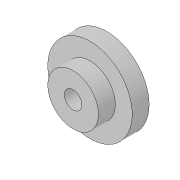
# Autodesk Inventor part: T-Spacer 3 of 32 inch
Saved by Autodesk Inventor 2018.3 (Build 223284000, 284)
## iProperties
Created: 2019-03-14
Part Number: T-Spacer 3 of 32 inch
Material: Generic
Document SubType Name: Modeling
Designer: aye06091
Mass: 0.797081 g
Surface Area: 6.96192 cm^2
Volume: 0.797081 cm^3
Density: 1 g/cm^3
Appearance: Default
Author: aye06091
Autodesk Inventor part; units mm, degrees
ref_plane "YZ Plane" through (0, 0, 0) normal (1, 0, 0) x (0, 1, 0)
ref_plane "XZ Plane" through (0, 0, 0) normal (0, 1, 0) x (-1, 0, 0)
ref_plane "XY Plane" through (0, 0, 0) normal (0, 0, 1) x (1, 0, 0)
sketch "Sketch4" plane through (0, 0, 0) normal (0, 0, 1) x (1, 0, 0)
  circle A0 centre (0, 0) radius 1.651
  circle A1 centre (0, 0) radius 4.7498
  dimension "d9" = 3.302
  dimension "d16" = 9.4996
  constraints: 2 centre point, 2 coincident
  measures "d9" diameter of A0
  measures "d16" diameter of A1
extrude "Extrusion4" add sketch "Sketch4" against normal blind 6.35
sketch "Sketch5" plane through (0, 0, -6.35) normal (0, 0, -1) x (-1, 0, 0)
  circle A0 centre (0, 0) radius 4.7498 projected
  circle A1 centre (0, 0) radius 7.9248
  dimension "d13" = 3.175
  constraints: 1 centre point, 1 coincident
  measures "d13" radial gap between concentric circles of A0 A1
extrude "Extrusion5" add sketch "Sketch5" against normal blind 3.175
equation "\"d14\" = 0.5 * d11"
equation "\"d11\" = 6.35"
body "Solid2"
